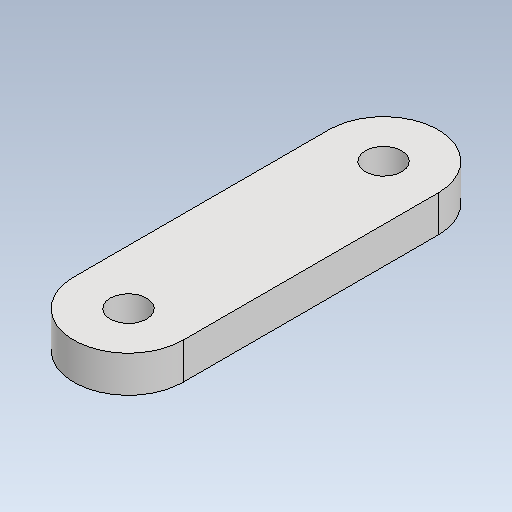
# Autodesk Inventor part: scissor-link
Saved by Autodesk Inventor 2025 (Build 290162000, 162)
## iProperties
Created: 2025-08-20
Part Number: scissor-link
Material: Generic
Document SubType Name: Modeling
Designer: HP
Density: 1 g/cm^3
Appearance: Default
Author: HP
Autodesk Inventor part; units mm, degrees
ref_plane "YZ Plane" through (0, 0, 0) normal (1, 0, 0) x (0, 1, 0)
ref_plane "XZ Plane" through (0, 0, 0) normal (0, 1, 0) x (-1, 0, 0)
ref_plane "XY Plane" through (0, 0, 0) normal (0, 0, 1) x (1, 0, 0)
sketch "Sketch1" plane through (0, 0, 0) normal (0, 1, 0) x (-1, 0, 0)
  line L0 (-7.5, 17.5) -> (7.5, 17.5) construction
  line L1 (7.5, 17.5) -> (7.5, -17.5)
  line L2 (7.5, -17.5) -> (-7.5, -17.5) construction
  line L3 (-7.5, -17.5) -> (-7.5, 17.5)
  line L4 (-7.5, 17.5) -> (7.5, -17.5) construction
  line L5 (7.5, 17.5) -> (-7.5, -17.5) construction
  circle A0 centre (0, 17.5) radius 2.5
  circle A1 centre (0, 17.5) radius 7.5
  circle A2 centre (0, -17.5) radius 2.5
  circle A3 centre (0, -17.5) radius 7.5
  point P0 (0, 0)
  point P1 (-7.5, 17.5)
  point P2 (-7.5, -17.5)
  dimension "d4" = 15
  dimension "d0" = 35
  dimension "d1" = 15
  dimension "d5" = 5
  dimension "d6" = 5
  constraints: 12 end point, 3 midpoint, 2 centre point, 2 coincident, 2 parallel, 1 horizontal, 1 perpendicular, 1 vertical alignment, 6 other
  measures "d0" distance between parallel lines of L2 L0
  measures "d1" distance between parallel lines of L3 L1
  measures "d5" diameter of A0
  measures "d6" diameter of A2
extrude "Extrusion1" add sketch "Sketch1" along normal blind 5
equation "\"d4\" = d1"
equation "\"d6\" = d5"
body "Solid1"
